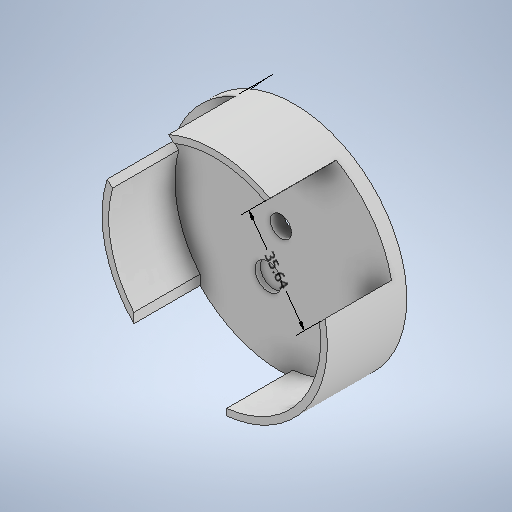
# Autodesk Inventor part: tryy2
Saved by Autodesk Inventor 2025.4 (Build 294407000, 407)
## iProperties
Created: 2026-04-05
Part Number: tryy2
Material: Generic
Document SubType Name: Modeling
Designer: Amir
Density: 1 g/cm^3
Appearance: Default
Author: Amir
Autodesk Inventor part; units mm, degrees
ref_plane "YZ Plane" through (0, 0, 0) normal (1, 0, 0) x (0, 1, 0)
ref_plane "XZ Plane" through (0, 0, 0) normal (0, 1, 0) x (-1, 0, 0)
ref_plane "XY Plane" through (0, 0, 0) normal (0, 0, 1) x (1, 0, 0)
sketch "Sketch1" plane through (0, 0, 0) normal (0, 0, 1) x (1, 0, 0)
  circle A0 centre (-0.0206, -3.7368) radius 40
  circle A1 centre (-0.0206, -3.7368) radius 42.5
  circle A2 centre (-0.0206, 1.2632) radius 4
  line L0 (-6.0206, 0.0132) -> (5.9794, 0.0132)
  line L1 (5.9794, 0.0132) -> (5.9794, 2.5132)
  line L2 (5.9794, 2.5132) -> (-6.0206, 2.5132)
  line L3 (-6.0206, 2.5132) -> (-6.0206, 0.0132)
  line L4 (-17.3849, 35.0541) -> (-15.3788, 33.1973)
  line L5 (-40.6108, 8.8603) -> (-38.5626, 6.9645)
  line L6 (19.021, 31.4401) -> (21.6473, 34.2375)
  line L7 (39.5419, 2.1626) -> (44.5969, 7.547)
  line L8 (4.4794, -43.4829) -> (4.4794, -45.9979)
  line L9 (-30.5206, -29.6164) -> (-30.5206, -33.3341)
  point P0 (0, 0)
  point P1 (-0.0206, -53.7368)
  point P2 (-0.0206, -9.5426)
  point P3 (-3.8203, 2.5132)
  point P4 (3.779, 2.5132)
  point P5 (3.779, 0.0132)
  point P6 (-3.8203, 0.0132)
  point P7 (-30.452, -29.697)
  point P8 (20.787, 33.3211)
  point P9 (41.6844, 4.4447)
  point P10 (-30.5206, -31.4752)
  dimension "d4" = 40
  dimension "d7" = 50
  dimension "d9" = 8
  dimension "d10" = 12
  dimension "d11" = 2.5
  dimension "d12" = 55
  dimension "d13" = 1.25
  dimension "d14" = 85
  dimension "d15" = 2.5
  dimension "d49" = 35
  dimension "d67" = 35
  dimension "d80" = 35
  constraints: 20 end point, 4 parallel, 4 point on circle, 2 centre point, 2 vertical, 1 coincident, 1 horizontal, 1 midpoint, 1 perpendicular, 1 vertical alignment, 9 other
  measures "d7" distance of A1.centre point (-0.021, -53.737)
  measures "d9" diameter of A2
  measures "d10" distance of L3.start L1.end
  measures "d11" distance of L1.end L0.end
  measures "d12" distance of point (-0.021, -53.737) A2.centre
  measures "d13" distance from line of A2.centre L0
  measures "d14" diameter of A1
  measures "d49" distance between parallel lines of L5 L4
  measures "d67" distance between parallel lines of L7 L6
  measures "d80" distance from line of point (-30.521, -31.475) L8
extrude "Extrusion1" add sketch "Sketch1" along normal blind 5 contours A0 | A0 L7 A1 L8 | A0 L6 A1 L7 | L8 A1 L9 A0 | A0 L4 A1 L6 | L9 A1 L5 A0 | A0 L5 A1 L4 | A2 L0 L2 | A2 L2 L1 L0 | L2 A2 | A2 L0 | A2 L0 L3 L2
extrude "Extrusion10" add sketch "Sketch1" along normal blind 30 contours A0 L7 A1 L8 | A0 L4 A1 L6 | L9 A1 L5 A0 | A2 L0 L2 | L2 A2 | A2 L0
extrude "Extrusion11" cut sketch "Sketch1" along normal blind 30 contours A2 L0 L2 | L2 A2 | A2 L0
sketch "Sketch2" plane through (0, 0, 5) normal (0, 0, 1) x (1, 0, 0)
  circle A0 centre (-0.0206, -3.7368) radius 42.5 projected
  circle A1 centre (-4.787, -17.567) radius 5
  point P0 (0, 0)
  dimension "d94" = 10
  constraints: 1 centre point
  measures "d94" diameter of A1
extrude "Extrusion12" cut sketch "Sketch2" against normal blind 2 contours A1
body "Solid1"
